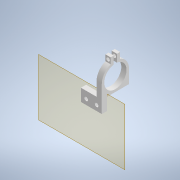
# Autodesk Inventor part: hopper motor holder
Saved by Autodesk Inventor 2022 (Build 260153000, 153)
## iProperties
Created: 2022-05-06
Part Number: hopper motor holder
Material: Generic
Document SubType Name: Modeling
Designer: efred
Density: 1 g/cm^3
Appearance: Default
Author: efred
Autodesk Inventor part; units mm, degrees
ref_plane "YZ Plane" through (0, 0, 0) normal (1, 0, 0) x (0, 1, 0)
ref_plane "XZ Plane" through (0, 0, 0) normal (0, 1, 0) x (-1, 0, 0)
ref_plane "XY Plane" through (0, 0, 0) normal (0, 0, 1) x (1, 0, 0)
ref_plane "Work Plane1" through (0, 0, 0) normal (0, 0, 1) x (1, 0, 0)
sketch "Sketch1" plane through (0, 0, 0) normal (0, 0, 1) x (1, 0, 0)
  circle A0 centre (25.75, 18) radius 1.7 projected
  circle A1 centre (-4.25, 18) radius 1.7 projected
  circle A2 centre (15.75, 18) radius 1.7 projected
  circle A3 centre (25.75, -18) radius 1.7 projected
  circle A4 centre (15.75, -18) radius 1.7 projected
  circle A5 centre (-4.25, -18) radius 1.7 projected
  line L0 (-12.45, 24.7) -> (32.45, 24.7) construction
  line L1 (-12.45, -24.7) -> (-12.45, 24.7) projected
  line L2 (-12.45, -24.7) -> (32.45, -24.7) projected
  line L3 (32.45, 24.7) -> (32.45, -24.7) projected
  circle A6 centre (-2.25, 0) radius 5.2 projected
  circle A7 centre (5.75, -18) radius 1.7 projected
  circle A8 centre (5.75, 18) radius 1.7 projected
  line L4 (10.75, 24.8) -> (30.75, 24.8)
  line L5 (30.75, 24.8) -> (30.75, 13)
  line L6 (30.75, 13) -> (10.75, 13)
  line L7 (10.75, 13) -> (10.75, 24.8)
  point P0 (0, 0)
  dimension "d0" = 5
  dimension "d1" = 5
  dimension "d2" = 5
  dimension "d3" = 0.1
  constraints: 8 end point, 2 parallel, 1 horizontal, 1 perpendicular
  measures "d0" distance from line of L6 A0.centre
  measures "d1" distance from line of A0.centre L5
  measures "d2" distance from line of L7 A2.centre
  measures "d3" distance between parallel lines of L0 L4
extrude "Extrusion1" add sketch "Sketch1" along normal blind 5 contours L4 L5 L6 L7
sketch "Sketch2" plane through (30.75, 13, 0) normal (1, 0, 0) x (0, 0, -1)
  line L0 (0, 11.8) -> (-5, 11.8) projected
  line L1 (-5, 11.8) -> (21, 11.8)
  line L2 (21, 11.8) -> (21, 37.8)
  line L3 (21, 37.8) -> (-5, 37.8)
  line L4 (-5, 37.8) -> (-5, 11.8)
  circle A0 centre (8, 24.8) radius 10.65
  circle A1 centre (8, 24.8) radius 13
  line L5 (6.5, 37.7132) -> (6.5, 35.3438)
  line L6 (9.5, 37.7132) -> (9.5, 35.3438)
  line L7 (8, 37.8) -> (8, 24.8) construction
  line L8 (6.5, 35.3438) -> (3.5, 35.3438)
  line L9 (3.5, 35.3438) -> (3.5, 42.7132)
  line L10 (3.5, 42.7132) -> (6.5, 42.7132)
  line L11 (6.5, 42.7132) -> (6.5, 35.3438)
  line L12 (12.5, 35.3438) -> (12.5, 42.7132)
  line L13 (12.5, 42.7132) -> (9.5, 42.7132)
  line L14 (9.5, 42.7132) -> (9.5, 35.3438)
  line L15 (9.5, 35.3438) -> (12.5, 35.3438)
  point P0 (0, -13)
  point P1 (21, 24.8)
  point P2 (-5, 24.8)
  point P3 (21, 24.8)
  point P4 (12.5, 36.9963)
  point P5 (3.5, 36.9963)
  dimension "d6" = 26
  dimension "d7" = 26
  dimension "d8" = 21.3
  dimension "d9" = 3
  dimension "d10" = 3
  dimension "d11" = 5
  constraints: 30 end point, 5 parallel, 4 point on circle, 3 symmetric about line, 2 centre point, 2 horizontal, 2 midpoint, 2 perpendicular, 2 vertical, 1 horizontal alignment, 1 tangent, 1 vertical alignment, 1 other
  measures "d6" distance of L2.end L3.end
  measures "d7" distance of L3.end L0.end
  measures "d8" diameter of A0
  measures "d9" distance between parallel lines of L5 L6
  measures "d10" distance between parallel lines of L9 L11
  measures "d11" distance of L10.end L5.start
extrude "Extrusion2" add sketch "Sketch2" against normal blind 5 contours L0 L4 A1 L1 | A1 L2 L1 | A1 L9 L8 A0 L15 L12 | L9 L3 L11 A1 | A1 L5 L8 L9 | L12 L15 L6 A1 | A1 L14 L3 L12 | L9 L10 L11 L3 | L3 L14 L13 L12
sketch "Sketch3" plane through (30.75, 49.9963, -3.5) normal (0, 0, 1) x (1, 0, 0)
  line L0 (0, 5.7169) -> (0, 0) projected
  line L1 (0, 5.7169) -> (-5, 5.7169) projected
  line L2 (-5, 0) -> (-5, 5.7169) projected
  line L3 (0, 0) -> (-5, 0) projected
  circle A0 centre (-2.5, 2.8584) radius 1.65
  point P0 (-30.75, -49.9963)
  point P1 (-5, 2.8584)
  point P2 (-2.5, 5.7169)
  dimension "d14" = 3.3
  constraints: 2 midpoint, 1 centre point, 1 horizontal alignment, 1 vertical alignment
  measures "d14" diameter of A0
extrude "Extrusion3" cut sketch "Sketch3" against normal through all contours A0
equation "\"d6\" = d7"
body "Solid1"
